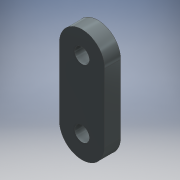
# Autodesk Inventor part: tracks_outer
Saved by Autodesk Inventor 2016 (Build 200138000, 138)
## iProperties
Created: 2016-11-08
Part Number: tracks_outer
Material: Generic
Document SubType Name: Modeling
Designer: hesaon
Density: 1 g/cm^3
Appearance: Default
Author: hesaon
Autodesk Inventor part; units mm, degrees
ref_plane "YZ Plane" through (0, 0, 0) normal (1, 0, 0) x (0, 1, 0)
ref_plane "XZ Plane" through (0, 0, 0) normal (0, 1, 0) x (-1, 0, 0)
ref_plane "XY Plane" through (0, 0, 0) normal (0, 0, 1) x (1, 0, 0)
sketch "Sketch1" plane through (0, 0, 0) normal (0, 1, 0) x (-1, 0, 0)
  line L0 (8.5, 0) -> (8.5, -12.7)
  line L1 (0, -12.7) -> (0, 0)
  circle A0 centre (4.25, 0) radius 1.4
  circle A1 centre (4.25, -12.7) radius 1.4
  arc A2 (8.5, 0) -> (0, 0) centre (4.25, 0) ccw
  arc A3 (0, -12.7) -> (8.5, -12.7) centre (4.25, -12.7) ccw
  dimension "d2" = 2.8
  dimension "d3" = 2.8
  dimension "pitch" = 12.7
  dimension "d7" = 4.25
  dimension "d10" = 4.25
  dimension "d11" = 12.7
  dimension "d12" = 0
  constraints: 4 centre point, 4 end point, 4 point on circle, 4 tangent, 1 coincident, 1 parallel, 1 vertical, 1 vertical alignment
  measures "d2" diameter of A0
  measures "d3" diameter of A1
  measures "pitch" distance of A1.centre A0.centre
  measures "d7" distance from line of L1 A0.centre
  measures "d10" radius of A2
  measures "d11" distance of L0.start L0.end
  measures "d12" vertical distance of point (0, 0) A0.centre
extrude "Extrusion1" add sketch "Sketch1" along normal blind 3
equation "\"d3\" = d2"
equation "\"d7\" = 0.5 * d0"
equation "\"d11\" = pitch"
equation "\"d0\" = 8.5"
body "Solid1"
